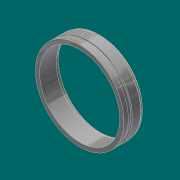
# Autodesk Inventor part: A1-19027-200-xx 32in Type B victaulic ring
Saved by Autodesk Inventor 2017.3 (Build 213256000, 256)
## iProperties
Created: 2013-12-16
Part Number: A1-19027-200-xx 32in Type B victaulic ring
Material: Steel, Mild
Document SubType Name: Modeling
Designer: Graeme_Van_Dongen
Density: 7.86 g/cm^3
Appearance: Steel
Description: 32" TYPE B VICTAULIC RING FOR STYLE 275 COUPLING, A105N, CUSTOM INVERTED B
Mass: 168590 g
Surface Area: 14074.5 cm^2
Volume: 21449.1 cm^3
Author: Graeme_Van_Dongen
Autodesk Inventor part; units mm, degrees
ref_plane "YZ Plane" through (0, 0, 0) normal (1, 0, 0) x (0, 1, 0)
ref_plane "XZ Plane" through (0, 0, 0) normal (0, 1, 0) x (-1, 0, 0)
ref_plane "XY Plane" through (0, 0, 0) normal (0, 0, 1) x (1, 0, 0)
sketch "Sketch1" plane through (0, 0, 0) normal (1, 0, 0) x (0, 1, 0)
  line L0 (396.875, 0) -> (396.875, 165.1)
  line L1 (396.875, 165.1) -> (438.15, 165.1)
  line L2 (438.15, 165.1) -> (438.15, 122.322)
  line L3 (438.15, 122.322) -> (425.45, 120.65)
  line L4 (425.45, 120.65) -> (425.45, 86.36)
  line L5 (425.45, 86.36) -> (438.15, 83.6026)
  line L6 (438.15, 83.6026) -> (438.15, 0)
  line L7 (0, -78.74) -> (0, 205.74) projected
  line L8 (431.8, -11.6105) -> (431.8, -23.2231)
  line L9 (431.8, -23.2231) -> (420.6875, -31.75)
  line L10 (420.6875, -31.75) -> (415.925, -31.75)
  line L11 (415.925, -31.75) -> (415.925, -38.1)
  line L12 (415.925, -38.1) -> (414.3375, -38.1)
  line L13 (414.3375, -38.1) -> (414.3375, -12.7)
  arc A0 (414.3375, -12.7) -> (401.6375, 0) centre (401.6375, -12.7) ccw
  line L14 (401.6375, 0) -> (396.875, 0)
  line L15 (438.15, 0) -> (435.5197, -2.6303)
  arc A1 (435.5197, -2.6303) -> (431.8, -11.6105) centre (444.5, -11.6105) ccw
  point P0 (0, 0)
  dimension "d0" = 396.875
  dimension "d5" = 165.1
  dimension "d13" = 425.45
  dimension "d14" = 438.15
  dimension "d16" = 44.45
  dimension "d17" = 34.29
  dimension "d18" = 7.5
  dimension "d19" = 12.25
  dimension "d32" = 431.8
  dimension "d33" = 11.1125
  dimension "d34" = 4.7625
  dimension "d35" = 1.5875
  dimension "d36" = 12.7
  dimension "d37" = 37.5
  dimension "d38" = 203.2
  dimension "d39" = 6.35
  dimension "d43" = 12.7
  dimension "d44" = 45
  dimension "d45" = 165.1
  constraints: 30 end point, 6 perpendicular, 4 point on circle, 4 tangent, 3 parallel, 2 centre point, 2 vertical, 1 collinear, 1 point on line
  measures "d0" distance from line of point (0, 0) L0
  measures "d5" distance of L0.start L0.end
  measures "d13" distance from line of point (0, 0) L4
  measures "d14" distance from line of point (0, 0) L6
  measures "d16" distance from line of L3.end L1
  measures "d17" distance of L3.end L4.end
  measures "d18" angle of L1 L3
  measures "d19" angle of L5 L1
  measures "d32" distance between parallel lines of L7 L8
  measures "d33" horizontal distance of L8.end L9.end
  measures "d34" distance of L9.end L10.end
  measures "d35" distance of L11.end L12.end
  measures "d36" radius of A0
  measures "d37" angle of L10 L9
  measures "d38" distance between parallel lines of L12 L1
  measures "d39" distance of L10.end L11.end
  measures "d43" radius of A1
  measures "d44" angle of L6 L15
  measures "d45" distance from line of L6.end L1
revolve "Revolution1" add sketch "Sketch1" angle 360 about axis through (0, 0, -10) along (0, 0, 1)
chamfer "Chamfer2" distance 0.7937 angle 45 1 edges at (0, -396.875, 0)
body "Solid1"
